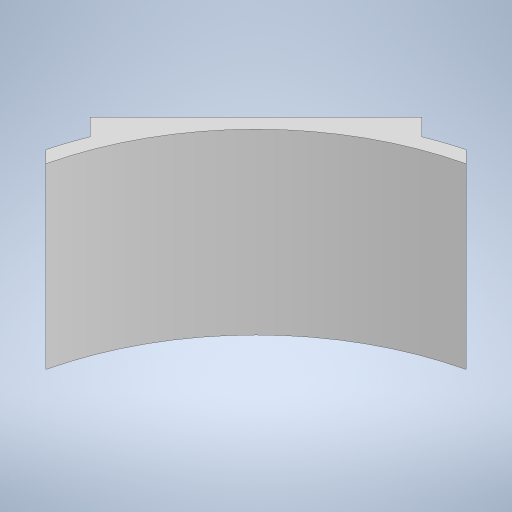
# Autodesk Inventor part: buttonholderscooterpart
Saved by Autodesk Inventor 2023 (Build 270158000, 158)
## iProperties
Created: 2023-10-25
Part Number: buttonholderscooterpart
Material: Generic
Document SubType Name: Modeling
Designer: zskus
Density: 1 g/cm^3
Appearance: Default
Author: zskus
Autodesk Inventor part; units mm, degrees
ref_plane "YZ Plane" through (0, 0, 0) normal (1, 0, 0) x (0, 1, 0)
ref_plane "XZ Plane" through (0, 0, 0) normal (0, 1, 0) x (-1, 0, 0)
ref_plane "XY Plane" through (0, 0, 0) normal (0, 0, 1) x (1, 0, 0)
sketch "Sketch1" plane through (0, 0, 0) normal (0, 1, 0) x (-1, 0, 0)
  circle A0 centre (0, 0) radius 24.13
  circle A1 centre (0, 0) radius 25.4
  line L0 (25.4, 0) -> (0, 0)
  line L1 (0, 0) -> (0, -25.4)
  point P0 (0, -24.13)
  point P1 (24.13, 0)
  dimension "d0" = 48.26
  dimension "d1" = 50.8
  constraints: 4 end point, 2 centre point, 2 coincident, 2 point on circle, 1 horizontal, 1 perpendicular
  measures "d0" diameter of A0
  measures "d1" diameter of A1
extrude "Extrusion1" add sketch "Sketch1" along normal blind 15.24 contours L0 A1 L1 A0 picked at (24.5627, -3.6738)
sketch "Sketch2" plane through (0, 15.24, 0) normal (0, 1, 0) x (1, 0, 0)
  line L0 (-25.0549, 10.8661) -> (-10.8661, 25.0549)
  arc A0 (0, 25.4) -> (-25.4, 0) centre (0, 0) ccw projected
  line L1 (0, 0) -> (-17.9605, 17.9605)
  line L2 (-25.0549, 10.8661) -> (-23.5944, 9.4056)
  line L3 (-10.8661, 25.0549) -> (-9.4056, 23.5944)
  point P0 (-17.9605, 17.9605)
  dimension "d4" = 20.066
  constraints: 8 end point, 4 point on circle, 1 midpoint, 1 parallel, 1 perpendicular, 1 tangent
  measures "d4" distance of L0.start L0.end
extrude "Extrusion2" add sketch "Sketch2" against normal up to surface (15.24 mm away)
sketch "Sketch3" plane through (0, 15.24, 0) normal (0, 1, 0) x (1, 0, 0)
  line L0 (-24.6957, 11.2253) -> (-11.2253, 24.6957) projected
  line L1 (-17.9605, 17.9605) -> (-8.9803, 26.9408)
  line L2 (-8.9803, 26.9408) -> (-5.2605, 23.221)
  line L3 (-5.2605, 23.221) -> (-23.221, 5.2605)
  line L4 (-23.221, 5.2605) -> (-26.9408, 8.9803)
  line L5 (-26.9408, 8.9803) -> (-17.9605, 17.9605)
  line L6 (-10.8661, 25.0549) -> (-25.0549, 10.8661) projected
  line L7 (-5.2605, 23.221) -> (3.175, 20.6375)
  line L8 (3.175, 20.6375) -> (3.175, 30.7046)
  line L9 (3.175, 30.7046) -> (-8.9803, 26.9408)
  line L10 (-26.9408, 8.9803) -> (-30.2776, -1.7961)
  line L11 (-30.2776, -1.7961) -> (-21.5572, -1.7961)
  line L12 (-21.5572, -1.7961) -> (-23.221, 5.2605)
  point P0 (0, 0)
  dimension "d7" = 12.7
  dimension "d8" = 12.7
  constraints: 22 end point, 5 perpendicular, 3 midpoint, 1 collinear, 1 point on line, 1 vertical
  measures "d7" distance from line of point (-17.961, 17.961) L2
  measures "d8" distance from line of point (-17.961, 17.961) L4
extrude "Extrusion3" cut sketch "Sketch3" against normal through all contours L4 L12 L11 L10 | L9 L8 L7 L2
equation "\"d8\" = d7"
body "Solid1"
